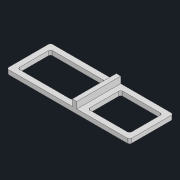
# Autodesk Inventor part: Part2
Saved by Autodesk Inventor 2022 (Build 260153000, 153)
## iProperties
Created: 2021-11-19
Part Number: Part2
Material: 一般
Document SubType Name: Modeling
Designer: Yuta Kage
Density: 1 g/cm^3
Appearance: 既定
Author: Yuta Kage
Autodesk Inventor part; units mm, degrees
ref_plane "YZ Plane" through (0, 0, 0) normal (1, 0, 0) x (0, 1, 0)
ref_plane "XZ Plane" through (0, 0, 0) normal (0, 1, 0) x (-1, 0, 0)
ref_plane "XY Plane" through (0, 0, 0) normal (0, 0, 1) x (1, 0, 0)
sketch "スケッチ1" plane through (0, 0, 0) normal (0, 1, 0) x (-1, 0, 0)
  line L0 (56, 20) -> (-56, 20)
  line L1 (-56, 20) -> (-56, -20)
  line L2 (-56, -20) -> (56, -20)
  line L3 (56, -20) -> (56, 20)
  line L4 (56, 20) -> (-56, -20) construction
  line L5 (-56, 20) -> (56, -20) construction
  point P0 (0, 0)
  dimension "d0" = 112
  dimension "d1" = 40
  constraints: 12 end point, 2 midpoint, 2 parallel, 1 horizontal, 1 perpendicular
  measures "d0" distance of L1.end L2.end
  measures "d1" distance of L0.end L1.end
extrude "押し出し1" add sketch "スケッチ1" along normal blind 10
sketch "スケッチ2" plane through (0, 10, 0) normal (0, 1, 0) x (1, 0, 0)
  line L0 (56, 20) -> (-56, 20) projected
  line L1 (-56, -20) -> (56, -20) projected
  line L2 (-56, 20) -> (4, 20)
  line L3 (4, 20) -> (4, -20)
  line L4 (4, -20) -> (-56, -20)
  line L5 (-56, -20) -> (-56, 20)
  line L6 (56, -20) -> (56, 20) projected
  line L7 (56, 20) -> (8, 20)
  line L8 (8, 20) -> (8, -20)
  line L9 (8, -20) -> (56, -20)
  line L10 (56, -20) -> (56, 20)
  point P0 (0, 0)
  point P1 (-56, -20)
  point P2 (4, 20)
  point P3 (8, 20)
  dimension "d4" = 60
  dimension "d5" = 48
  constraints: 16 end point, 4 parallel, 2 horizontal, 2 perpendicular, 2 point on line
  measures "d4" distance between parallel lines of L5 L3
  measures "d5" distance between parallel lines of L6 L8
extrude "押し出し2" cut sketch "スケッチ2" against normal blind 6 contours L6 L1 L8 L0 | L3 L1 L5 L0
fillet "フィレット1" radius 2 4 edges at (-56, 2, 20) (-56, 2, -20) (56, 2, -20) (56, 2, 20)
sketch "スケッチ3" plane through (0, 4, 0) normal (0, 1, 0) x (1, 0, 0)
  line L0 (-51, -15) -> (-1, -15)
  line L1 (-1, -15) -> (-1, 15)
  line L2 (-1, 15) -> (-51, 15)
  line L3 (-51, 15) -> (-51, -15)
  line L4 (-51, -15) -> (-1, 15) construction
  line L5 (-1, -15) -> (-51, 15) construction
  line L6 (13, -15) -> (51, -15)
  line L7 (51, -15) -> (51, 15)
  line L8 (51, 15) -> (13, 15)
  line L9 (13, 15) -> (13, -15)
  line L10 (13, -15) -> (51, 15) construction
  line L11 (51, -15) -> (13, 15) construction
  line L12 (8, 20) -> (54, 20) projected
  line L13 (56, 18) -> (56, -18) projected
  line L14 (54, -20) -> (8, -20) projected
  line L15 (8, -20) -> (8, 20) projected
  line L16 (-54, 20) -> (4, 20) projected
  line L17 (-56, -18) -> (-56, 18) projected
  line L18 (4, -20) -> (-54, -20) projected
  line L19 (4, 20) -> (4, -20) projected
  point P0 (0, 0)
  point P1 (-26, 0)
  point P2 (32, 0)
  dimension "d9" = 5
  dimension "d10" = 5
  dimension "d11" = 5
  dimension "d12" = 5
  dimension "d13" = 5
  dimension "d14" = 5
  dimension "d15" = 5
  dimension "d16" = 5
  constraints: 24 end point, 4 midpoint, 4 parallel, 2 horizontal, 2 perpendicular
  measures "d9" distance between parallel lines of L12 L8
  measures "d10" distance between parallel lines of L13 L7
  measures "d11" distance between parallel lines of L14 L6
  measures "d12" distance between parallel lines of L15 L9
  measures "d13" distance between parallel lines of L16 L2
  measures "d14" distance between parallel lines of L17 L3
  measures "d15" distance between parallel lines of L18 L0
  measures "d16" distance between parallel lines of L19 L1
extrude "押し出し3" cut sketch "スケッチ3" against normal blind 6
fillet "フィレット2" radius 2 8 edges at (-51, 2, -15) (-1, 2, -15) (-51, 2, 15) (-1, 2, 15) (13, 2, -15) (51, 2, -15) (13, 2, 15) (51, 2, 15)
equation "\"d10\" = d9"
equation "\"d11\" = d9"
equation "\"d12\" = d9"
equation "\"d13\" = d9"
equation "\"d14\" = d9"
equation "\"d15\" = d9"
equation "\"d16\" = d9"
